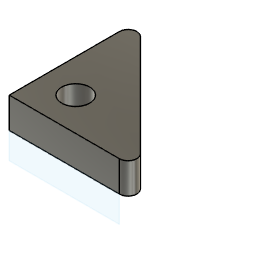
M3 spacer (Autodesk Fusion 360 design; units mm, degrees)
Autodesk Fusion 360 part; units mm, degrees
imported_body "Base Feature1" makes body 1
sketch "Sketch1" plane through (0, -3.8, 0) normal (0, -1, 0) x (1, 0, 0)
  line L0 (8.7858, 0) -> (8.7858, 3)
  line L1 (8.7858, 3) -> (-3.8, 3)
  line L2 (-3.8, 3) -> (-3.8, 0)
  line L3 (-3.8, 0) -> (8.7858, 0)
sketch "Sketch2" plane through (0, 0, 3) normal (0, 0, 1) x (-1, 0, 0)
  line L0 (-3.5134, -0.9414) -> (-2.572, 2.572)
  line L1 (-2.572, 2.572) -> (0.9414, 3.5134)
  line L2 (0.9414, 3.5134) -> (3.5134, 0.9414)
  line L3 (3.5134, 0.9414) -> (2.572, -2.572)
  line L4 (2.572, -2.572) -> (-0.9414, -3.5134)
  line L5 (-0.9414, -3.5134) -> (-3.5134, -0.9414)
  line L6 (-9.4929, 2.0929) -> (2.0929, -9.4929)
  arc A0 (2.0929, -9.4929) -> (3.8, -8.7858) centre (2.8, -8.7858) ccw
  line L7 (3.8, -8.7858) -> (3.8, 3.8)
  line L8 (3.8, 3.8) -> (-8.7858, 3.8)
  arc A1 (-8.7858, 3.8) -> (-9.4929, 2.0929) centre (-8.7858, 2.8) ccw
  line L9 (3.8, 3.8) -> (3.8, -8.7858)
  line L10 (3.8, 3.8) -> (-8.7858, 3.8)
  line L11 (-9.4929, 2.0929) -> (2.0929, -9.4929)
  line L12 (2.0929, -9.4929) -> (3.8, -11.2)
  line L13 (3.8, -11.2) -> (3.8941, -11.1059)
  line L14 (3.8, -8.7858) -> (3.8, -11.2)
  line L15 (-8.7858, 3.8) -> (-11.5, 3.8)
  line L16 (-9.4929, 2.0929) -> (-11.2, 3.8)
  circle A2 centre (0, 0) radius 1.6
  dimension "d1" = 3.2
  constraint coincident L7.end L8.start
  constraint coincident A0.end L7.start
  constraint coincident L8.end A1.start
  constraint coincident L6.start A1.end
  constraint coincident L6.end A0.start
  constraint tangent A0 L12
  constraint perpendicular L11 L13
  constraint tangent A0 L14
  constraint tangent A1 L15
  constraint coincident L15 L16.end
  constraint tangent A1 L16
  constraint coincident A2.centre origin
  measures "d1" diameter of A2
extrude "Extrude1" add sketch "Sketch2" along normal blind 3.5 separate body contours L0 L1 L2 L3 L4 L5 | L6 A0 L7 L8 A1 L9 L10 L11 makes body 2
delete_body "RemoveBody1" bodies 1
